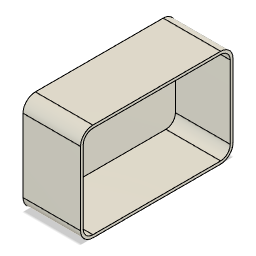
support inf v3 (Autodesk Fusion 360 design; units mm, degrees)
Autodesk Fusion 360 part; units mm, degrees
sketch "Esquisse1" plane through (0, 0, 0) normal (1, 0, 0) x (0, 0, -1)
  line L0 (166.9054, -107.1527) -> (-0.0946, -107.1527)
  circle A0 centre (13.4054, -93.6527) radius 13.5
  line L1 (-0.0946, -107.1527) -> (-0.0946, -0.1527)
  circle A1 centre (13.4054, -13.6527) radius 13.5
  line L2 (-0.0946, -0.1527) -> (166.9054, -0.1527)
  circle A2 centre (153.4054, -13.6527) radius 13.5
  line L3 (166.9054, -0.1527) -> (166.9054, -107.1527)
  circle A3 centre (153.4054, -93.6527) radius 13.5
  dimension "d44" = 107
  dimension "d45" = 167
  dimension "d24" = 27
  dimension "d25" = 27
  dimension "d26" = 27
  dimension "d27" = 27
  constraint horizontal L2
  constraint vertical L3
  constraint horizontal L0
  constraint vertical L1
  measures "d44" distance of L2.end L0.start
  measures "d45" distance of L2.end L1.end
  measures "d24" diameter of A2
  measures "d25" diameter of A1
  measures "d26" diameter of A3
  measures "d27" diameter of A0
extrude "Extrusion3" add sketch "Esquisse1" along normal blind 3 contours L0 A0 L1 A1 L2 A2 L3 A3 | A3 | A0 | A2 | A1
sketch "Esquisse3" plane through (3, 0, 0) normal (1, 0, 0) x (0, 0, -1)
  arc A0 (13.4054, -0.1527) -> (-0.0946, -13.6527) centre (13.4054, -13.6527) ccw
  line L0 (-0.0946, -13.6527) -> (-0.0946, -93.6527)
  arc A1 (-0.0946, -93.6527) -> (13.4054, -107.1527) centre (13.4054, -93.6527) ccw
  line L1 (13.4054, -107.1527) -> (153.4054, -107.1527)
  arc A2 (153.4054, -107.1527) -> (166.9054, -93.6527) centre (153.4054, -93.6527) ccw
  line L2 (166.9054, -93.6527) -> (166.9054, -13.6527)
  arc A3 (166.9054, -13.6527) -> (153.4054, -0.1527) centre (153.4054, -13.6527) ccw
  line L3 (153.4054, -0.1527) -> (13.4054, -0.1527)
  line L4 (13.4054, -0.1527) -> (13.4054, -107.1527)
  line L5 (-0.0946, -13.6527) -> (166.9054, -13.6527)
  line L6 (153.4054, -0.1527) -> (153.4054, -107.1527)
  line L7 (166.9054, -93.6527) -> (-0.0946, -93.6527)
  line L8 (13.4054, -3.1527) -> (153.4054, -3.1527)
  line L9 (163.9054, -13.6527) -> (163.9054, -93.6527)
  line L10 (153.4054, -104.1527) -> (13.4054, -104.1527)
  line L11 (2.9054, -93.6527) -> (2.9054, -13.6527)
  line L12 (-0.0946, -0.1527) -> (166.9054, -0.1527)
  line L13 (-0.0946, -107.1527) -> (-0.0946, -0.1527)
  line L14 (166.9054, -107.1527) -> (-0.0946, -107.1527)
  line L15 (166.9054, -0.1527) -> (166.9054, -107.1527)
  arc A4 (13.4054, -3.1527) -> (2.9054, -13.6527) centre (13.4054, -13.6527) ccw
  arc A5 (163.9054, -13.6527) -> (153.4054, -3.1527) centre (153.4054, -13.6527) ccw
  arc A6 (2.9054, -93.6527) -> (13.4054, -104.1527) centre (13.4054, -93.6527) ccw
  arc A7 (153.4054, -104.1527) -> (163.9054, -93.6527) centre (153.4054, -93.6527) ccw
  dimension "d52" = 3
  dimension "d53" = 3
  dimension "d54" = 3
  dimension "d55" = 3
  constraint coincident A0.start L3.end
  constraint coincident A1.end L1.start
  constraint coincident A0.end L0.start
  constraint coincident L2.end A3.start
  constraint coincident A3.end L3.start
  constraint coincident L1.end A2.start
  constraint coincident A2.end L2.start
  constraint coincident L0.end A1.start
  constraint coincident L4 L8.start
  constraint coincident L6 L8.end
  constraint perpendicular L6 L8
  constraint coincident L5 L9.start
  constraint coincident L7 L9.end
  constraint perpendicular L7 L9
  constraint coincident L6 L10.start
  constraint coincident L4 L10.end
  constraint perpendicular L4 L10
  constraint coincident L7 L11.start
  constraint coincident L5 L11.end
  constraint perpendicular L5 L11
  constraint coincident A0.centre A4.centre
  constraint coincident A1.centre A6.centre
  measures "d52" distance of L8 L12
  measures "d53" distance of L11 L13
  measures "d54" distance of L10 L14
  measures "d55" distance of L9 L15
extrude "Extrusion4" add sketch "Esquisse3" along normal blind 60 contours A0 L4 L5 A4 | L3 L4 L6 L8 L12 | L0 L5 L7 L11 L13 | A3 L5 L6 A5 | A1 L4 L7 A6 | L2 L5 L7 L9 L15 | L1 L4 L6 L10 L14 | A2 L6 L7 A7
equation "d10 = largEntrePied + diaPiedBois"
equation "d11 = longEntrePied + diaPiedBois"
equation "d12 = diaPiedBois"
equation "d13 = diaExtPiedBois / 2"
equation "d14 = diaExtPiedBois / 2"
equation "d15 = diaPiedBois"
equation "d16 = diaPiedBois"
equation "d17 = diaPiedBois"
equation "d18 = diaExtPiedBois / 2"
equation "d44 = largEntrePied + diaExtPiedBois"
equation "d45 = longEntrePied + diaExtPiedBois"
equation "d24 = diaPiedBois + 5 mm"
equation "d25 = diaPiedBois + 5 mm"
equation "d26 = diaPiedBois + 5 mm"
equation "d27 = diaPiedBois + 5 mm"
